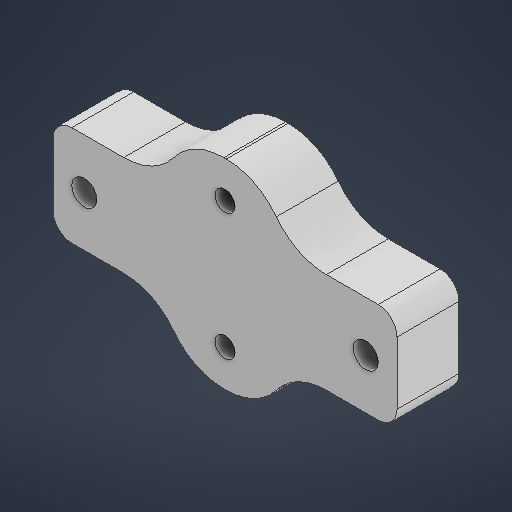
# Autodesk Inventor part: 14,9mm
Saved by Autodesk Inventor 2026.1 (Build 301233020, 233B)
## iProperties
Created: 2025-11-27
Part Number: 14,9mm
Material: Genérico
Document SubType Name: Modeling
Designer: Lucas David
Density: 1 g/cm^3
Appearance: Padrão
Author: Lucas David
Autodesk Inventor part; units mm, degrees
ref_plane "YZ Plane" through (0, 0, 0) normal (1, 0, 0) x (0, 1, 0)
ref_plane "XZ Plane" through (0, 0, 0) normal (0, 1, 0) x (-1, 0, 0)
ref_plane "XY Plane" through (0, 0, 0) normal (0, 0, 1) x (1, 0, 0)
sketch "Esboço1" plane through (0, 0, 0) normal (0, 0, 1) x (1, 0, 0)
  line L0 (-27.5, -8) -> (27.5, -8)
  line L1 (27.5, -8) -> (27.5, 8)
  line L2 (27.5, 8) -> (-27.5, 8)
  line L3 (-27.5, 8) -> (-27.5, -8)
  line L4 (-27.5, -8) -> (27.5, 8) construction
  line L5 (27.5, -8) -> (-27.5, 8) construction
  circle A0 centre (-22.5, 0) radius 1.6
  circle A1 centre (22.5, 0) radius 1.6
  line L6 (10, -16) -> (-10, -16)
  line L7 (-10, -16) -> (-10, 16)
  line L8 (-10, 16) -> (10, 16)
  line L9 (10, 16) -> (10, -16)
  line L10 (10, -16) -> (-10, 16) construction
  line L11 (-10, -16) -> (10, 16) construction
  circle A2 centre (0, 10.125) radius 1.6
  circle A3 centre (0, -10.125) radius 1.6
  point P0 (0, 0)
  point P1 (-10, -8)
  point P2 (10, -8)
  point P3 (10, 8)
  point P4 (-10, 8)
  dimension "d0" = 45
  dimension "d1" = 5
  dimension "d2" = 5
  dimension "d3" = 8
  dimension "d4" = 8
  dimension "d5" = 8
  dimension "d6" = 3.2
  dimension "d7" = 3.2
  dimension "d13" = 32
  dimension "d14" = 20
  dimension "d15" = 10.125
  dimension "d16" = 10.125
  dimension "d17" = 3.2
  dimension "d18" = 3.2
  dimension "d19" = 10
  dimension "d20" = 10
  constraints: 24 end point, 4 centre point, 4 midpoint, 4 parallel, 2 horizontal, 2 perpendicular
  measures "d0" distance of A1.centre A0.centre
  measures "d1" distance from line of L3 A0.centre
  measures "d2" distance from line of L1 A1.centre
  measures "d3" distance from line of L0 A0.centre
  measures "d4" distance from line of L2 A0.centre
  measures "d5" distance from line of L2 A1.centre
  measures "d6" diameter of A1
  measures "d7" diameter of A0
  measures "d13" distance between parallel lines of L6 L8
  measures "d14" distance between parallel lines of L9 L7
  measures "d15" distance of point (0, 0) A3.centre
  measures "d16" distance of point (0, 0) A2.centre
  measures "d17" diameter of A2
  measures "d18" diameter of A3
  measures "d19" distance from line of L7 A3.centre
  measures "d20" distance from line of L7 A2.centre
extrude "Extrusão1" add sketch "Esboço1" along normal blind 9.9 contours L3 L2 L7 L0 | L7 L2 L9 L0 | L0 L9 L6 L7 | L9 L2 L1 L0 | L7 L8 L9 L2 | A0 | A1 | A2 | A3
extrude "Extrusão2" cut sketch "Esboço1" along normal blind 14.9 contours A0 | A1
extrude "Extrusão3" cut sketch "Esboço1" against normal blind 8.9 from surface at 9.9 contours A2 | A3
fillet "Arredondamento1" radius 10 4 edges at (-10, -16, 4.95) (10, -16, 4.95) (-10, 16, 4.95) (10, 16, 4.95)
sketch "Esboço2" plane through (0, 0, 9.9) normal (0, 0, 1) x (1, 0, 0)
  arc A0 (0.202, -16) -> (10, -8) centre (0.202, -6) ccw projected
  line L0 (0.202, -16) -> (-0.202, -16) projected
  arc A1 (-10, -8) -> (-0.202, -16) centre (-0.202, -6) ccw projected
  line L1 (-10, -8) -> (-27.5, -8) projected
  line L2 (-27.5, -8) -> (-27.5, 8) projected
  line L3 (-27.5, 8) -> (-10, 8) projected
  arc A2 (-0.202, 16) -> (-10, 8) centre (-0.202, 6) ccw projected
  line L4 (-0.202, 16) -> (0.202, 16) projected
  arc A3 (10, 8) -> (0.202, 16) centre (0.202, 6) ccw projected
  line L5 (10, 8) -> (27.5, 8) projected
  line L6 (27.5, 8) -> (27.5, -8) projected
  line L7 (27.5, -8) -> (10, -8) projected
  circle A4 centre (0, 10.125) radius 1.6 projected
  circle A5 centre (0, -10.125) radius 1.6 projected
  circle A6 centre (22.5, 0) radius 1.6 projected
  circle A7 centre (-22.5, 0) radius 1.6 projected
  circle A8 centre (-22.5, 0) radius 2
  circle A9 centre (22.5, 0) radius 2
  point P0 (0, 0)
  dimension "d28" = 4
  dimension "d29" = 4
  constraints: 2 centre point
  measures "d28" diameter of A8
  measures "d29" diameter of A9
extrude "Extrusão4" cut sketch "Esboço2" against normal blind 8 contours A7 | A8 | A9
fillet "Arredondamento2" radius 10 4 edges at (10, -8, 4.95) (-10, -8, 4.95) (-10, 8, 4.95) (10, 8, 4.95)
fillet "Arredondamento3" radius 3 4 edges at (-27.5, -8, 4.95) (-27.5, 8, 4.95) (27.5, 8, 4.95) (27.5, -8, 4.95)
